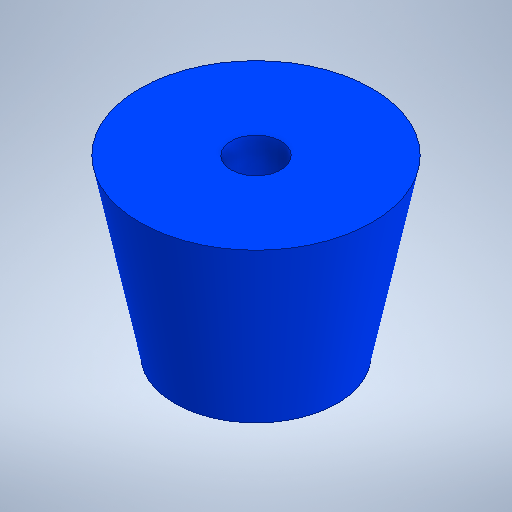
# Autodesk Inventor part: PrinterFeet
Saved by Autodesk Inventor 2025.2 (Build 292293000, 293)
## iProperties
Created: 2025-09-16
Part Number: PrinterFeet
Material: Generic
Document SubType Name: Modeling
Designer: Simon
Density: 1 g/cm^3
Appearance: Default(1)
Author: Simon
Autodesk Inventor part; units mm, degrees
ref_plane "YZ Plane" through (0, 0, 0) normal (1, 0, 0) x (0, 1, 0)
ref_plane "XZ Plane" through (0, 0, 0) normal (0, 1, 0) x (-1, 0, 0)
ref_plane "XY Plane" through (0, 0, 0) normal (0, 0, 1) x (1, 0, 0)
sketch "Sketch1" plane through (0, 0, 0) normal (1, 0, 0) x (0, 1, 0)
  line L0 (0, 0) -> (0, 7)
  line L1 (0, 7) -> (15, 7)
  line L2 (15, 7) -> (15, 10)
  line L3 (15, 10) -> (0, 7)
  line L4 (0, 0) -> (0, 2.15)
  line L5 (15, 7) -> (15, 0)
  line L6 (15, 0) -> (0, 0)
  line L7 (15, 0) -> (4, 0)
  line L8 (4, 0) -> (4, 4)
  line L9 (4, 4) -> (0, 4)
  line L10 (0, 2.15) -> (15, 2.15)
  point P0 (4, 2.15)
  dimension "d0" = 7
  dimension "d1" = 15
  dimension "d2" = 3
  dimension "d3" = 2.15
  dimension "d4" = 11
  dimension "d5" = 4
  constraints: 22 end point, 6 perpendicular, 4 point on line, 2 vertical
  measures "d0" distance of L0.start L0.end
  measures "d1" distance of L0.end L1.end
  measures "d2" distance of L1.end L2.end
  measures "d3" distance of L0.start L4.end
  measures "d4" distance of L5.end L7.end
  measures "d5" distance of L7.end L8.end
revolve "Revolution1" add sketch "Sketch1" angle 360 about axis through (0, 15, 0) along (0, -1, 0) contours L0 L1 L5 L10 L8 L9 | L3 L2 L1
body "Solid1"
